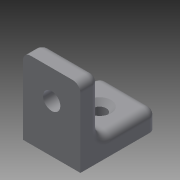
# Autodesk Inventor part: escuadra
Saved by Autodesk Inventor 2015 SP1 (Build 190203100, 203)
## iProperties
Created: 2015-04-01
Part Number: escuadra
Material: Generic
Document SubType Name: Modeling
Designer: pc
Density: 1 g/cm^3
Appearance: Default
Author: pc
Autodesk Inventor part; units mm, degrees
ref_plane "YZ Plane" through (0, 0, 0) normal (1, 0, 0) x (0, 1, 0)
ref_plane "XZ Plane" through (0, 0, 0) normal (0, 1, 0) x (-1, 0, 0)
ref_plane "XY Plane" through (0, 0, 0) normal (0, 0, 1) x (1, 0, 0)
sketch "Sketch1" plane through (0, 0, 0) normal (1, 0, 0) x (0, 1, 0)
  line L0 (0, 0) -> (0, 23.2432)
  line L1 (0, 23.2432) -> (0, 0)
  line L2 (0, 0) -> (17.5676, 0)
  line L3 (0, 0) -> (0, -18.1081)
  line L4 (0, 0) -> (-14.0541, 0)
  line L5 (-2.5, 10) -> (-2.5, -10)
  line L6 (-2.5, -10) -> (17.5, -10)
  line L7 (17.5, -10) -> (17.5, -5)
  line L8 (17.5, -5) -> (2.5, -5)
  line L9 (2.5, -5) -> (2.5, 10)
  line L10 (2.5, 10) -> (-2.5, 10)
  dimension "d0" = 20
  dimension "d1" = 5
  dimension "d2" = 5
  dimension "d3" = 20
  constraints: 22 end point, 5 perpendicular, 3 vertical, 2 horizontal, 2 symmetric about line, 1 collinear
  measures "d0" distance of L5.start L5.end
  measures "d1" distance of L9.end L5.start
  measures "d2" distance of L6.end L7.end
  measures "d3" distance of L5.end L6.end
extrude "Extrusion1" add sketch "Sketch1" along normal blind 15
sketch "Sketch2" plane through (0, -2.5, -10) normal (0, -1, 0) x (1, 0, 0)
  line L0 (0, 20) -> (0, 0) projected
  line L1 (0, 0) -> (15, 0) projected
  line L2 (15, 20) -> (15, 0) projected
  line L3 (0, 20) -> (15, 20) projected
  circle A0 centre (7.5, 12.5) radius 2.25
  point P0 (0, 10)
  dimension "d6" = 4.5
  dimension "d7" = 12.5
  constraints: 1 centre point
  measures "d6" diameter of A0
  measures "d7" distance from line of L1 A0.centre
extrude "Extrusion2" cut sketch "Sketch2" against normal through all contours A0
sketch "Sketch3" plane through (0, 2.5, -5) normal (0, 0, 1) x (1, 0, 0)
  line L0 (0, 15) -> (0, 0) projected
  line L1 (0, 0) -> (15, 0) projected
  line L2 (15, 15) -> (15, 0) projected
  line L3 (0, 15) -> (15, 15) projected
  circle A0 centre (7.5, 7.5) radius 1.75
  point P0 (0, -2.5)
  dimension "d10" = 3.5
  constraints: 1 centre point
  measures "d10" diameter of A0
extrude "Extrusion3" cut sketch "Sketch3" against normal through all contours A0
chamfer "Chamfer1" distance 1.25 angle 45 1 edges at (5.75, 10, -5)
chamfer "Chamfer2" distance 1.5 angle 45 1 edges at (5.25, 2.5, 2.5)
fillet "Fillet1" radius 3 1 edges at (7.5, 2.5, -5)
fillet "Fillet2" radius 2 10 edges at (15, 0, 10) (15, 11.5, -5) (15, 2.5, 4) (15, 17.5, -7.5) (7.5, 2.5, 10) (0, 11.5, -5) (0, 2.5, 4) (7.5, 17.5, -5) (0, 0, 10) (0, 17.5, -7.5)
body "Solid1"
